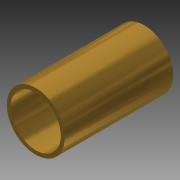
# Autodesk Inventor part: am-2243
Saved by Autodesk Inventor 2013 (Build 170138000, 138)
## iProperties
Category: Drive Base Kit
Company: Autodesk Inc.
Created: 2012-12-21
Part Number: am-2243
Material: Brass, Soft Yellow
Document SubType Name: Modeling
Designer: Autodesk Inc.
Density: 9.08119 g/cm^3
Catalog Web Link: http://www.andymark.com/product-p/am-2243.htm
Vendor: AndyMark Inc.
Mass: 4.53592 g
Surface Area: 14.0416 cm^2
Volume: 0.499486 cm^3
Author: Autodesk Inc.
Autodesk Inventor part; units mm, degrees
ref_plane "YZ Plane" through (0, 0, 0) normal (1, 0, 0) x (0, 1, 0)
ref_plane "XZ Plane" through (0, 0, 0) normal (0, 1, 0) x (-1, 0, 0)
ref_plane "XY Plane" through (0, 0, 0) normal (0, 0, 1) x (1, 0, 0)
sketch "Sketch1" plane through (0, 0, 0) normal (0, 0, 1) x (1, 0, 0)
  circle A0 centre (0, 0) radius 4.8133
  circle A1 centre (0, 0) radius 5.5499
  dimension "d0" = 9.6266
  dimension "d2" = 11.0998
  constraints: 2 centre point, 2 coincident
  measures "d0" diameter of A0
  measures "d2" diameter of A1
extrude "Extrusion1" add sketch "Sketch1" against normal blind 20.828
body "Solid1"
